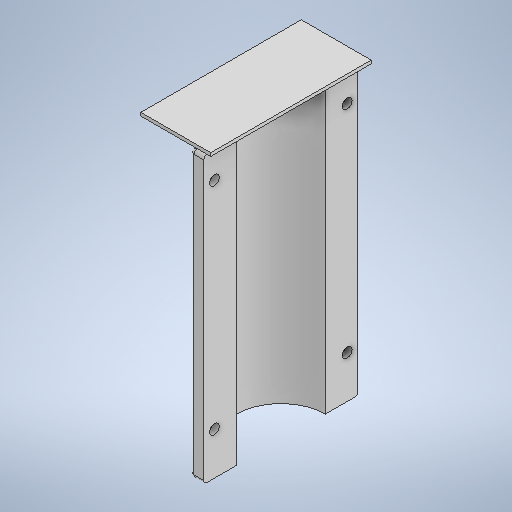
# Autodesk Inventor part: arm-2-2
Saved by Autodesk Inventor 2025.2 (Build 292293000, 293)
## iProperties
Created: 2025-02-07
Part Number: arm-2-2
Material: 一般
Document SubType Name: Modeling
Designer: mahhy
Density: 1 g/cm^3
Appearance: 既定
Author: mahhy
## iProperties of the stored document arm-2-2_3D プリント.ipt
Created: 2025-02-09
Part Number: arm-2-2_3D プリント
Material: 一般
Document SubType Name: Modeling
Designer: mahhy
Density: 1 g/cm^3
Appearance: 既定
Author: mahhy
Autodesk Inventor part; units mm, degrees
ref_plane "YZ Plane" through (0, 0, 0) normal (1, 0, 0) x (0, 1, 0)
ref_plane "XZ Plane" through (0, 0, 0) normal (0, 1, 0) x (-1, 0, 0)
ref_plane "XY Plane" through (0, 0, 0) normal (0, 0, 1) x (1, 0, 0)
sketch "スケッチ1" plane through (0, 0, 0) normal (0, 1, 0) x (-1, 0, 0)
  line L0 (0, 0) -> (20, 0)
  line L1 (20, 0) -> (20, -40)
  line L2 (20, -40) -> (0, -40)
  line L3 (0, -40) -> (0, 0)
  circle A0 centre (0, -20) radius 13.6
  circle A1 centre (0, -20) radius 17.5
  line L4 (0, -6.4) -> (4, -6.4)
  line L5 (4, -6.4) -> (4, 3.6)
  line L6 (4, 3.6) -> (0, 3.6)
  line L7 (0, 3.6) -> (0, -6.4)
  line L8 (0, -33.6) -> (4, -33.6)
  line L9 (4, -33.6) -> (4, -43.6)
  line L10 (4, -43.6) -> (0, -43.6)
  line L11 (0, -43.6) -> (0, -33.6)
  point P0 (0, -6.4)
  point P1 (0, -33.6)
  point P2 (4, -37.0367)
  point P3 (4, -2.9633)
  dimension "d0" = 20
  dimension "d1" = 40
  dimension "d2" = 27.2
  dimension "d3" = 35
  dimension "d4" = 4
  dimension "d5" = 10
  dimension "d6" = 4
  dimension "d7" = 10
  constraints: 24 end point, 6 parallel, 3 horizontal, 3 perpendicular, 2 centre point, 2 point on circle, 1 coincident, 1 midpoint
  measures "d0" distance of L1.end L2.end
  measures "d1" distance of L0.end L1.end
  measures "d2" diameter of A0
  measures "d3" diameter of A1
  measures "d4" distance of L6.end L5.end
  measures "d5" distance of L5.end L4.end
  measures "d6" distance of L9.end L10.end
  measures "d7" distance of L8.end L9.end
extrude "押し出し1" add sketch "スケッチ1" along normal blind 87 contours L7 L6 L5 L0 | L0 L5 A1 L3 | A1 L5 L4 L3 | A1 L9 L8 A0 L4 L5 | A1 L9 L2 L3 | L3 L8 L9 A1 | L2 L9 L10 L11
sketch "スケッチ2" plane through (-4, 0, -43.6) normal (-1, 0, 0) x (0, 0, 1)
  line L0 (0, 87) -> (6.5633, 87) projected
  line L1 (40.6367, 87) -> (47.2, 87) projected
  line L2 (40.6367, 0) -> (47.2, 0) projected
  line L3 (0, 0) -> (6.5633, 0) projected
  point P0 (43.6, 0)
  point P1 (3.2816, 13)
  point P2 (3.2816, 79)
  point P3 (43.9184, 79)
  point P4 (43.9184, 13)
  point P5 (3.2816, 87)
  point P6 (43.9184, 87)
  point P7 (43.9184, 0)
  point P8 (3.2816, 0)
  dimension "d10" = 0
  dimension "d11" = 8
  dimension "d12" = 0
  dimension "d13" = 8
  dimension "d14" = 0
  dimension "d15" = 0
  dimension "d16" = 13
  dimension "d17" = 13
  constraints: 4 midpoint
  measures "d10" horizontal distance of point (3.282, 87) point (3.282, 79)
  measures "d11" distance from line of L0 point (3.282, 79)
  measures "d12" horizontal distance of point (43.918, 87) point (43.918, 79)
  measures "d13" distance from line of L1 point (43.918, 79)
  measures "d14" horizontal distance of point (43.918, 0) point (43.918, 13)
  measures "d15" horizontal distance of point (3.282, 0) point (3.282, 13)
  measures "d16" vertical distance of L3.start point (3.282, 13)
  measures "d17" vertical distance of L2.end point (43.918, 13)
hole "穴1" at (-4, 13, -40.3184) at (-4, 79, -40.3184) at (-4, 79, 0.3184) at (-4, 13, 0.3184) direction (1, 0, 0) diameter 3 end through all
fillet "フィレット1" radius 1 14 edges at (-4, 87, 0.3184) (-17.5, 87, -20) (-4, 87, -40.3184) (-2, 87, -43.6) (-2, 87, 3.6) (-4, 43.5, 3.6) (-4, 0, 0.3184) (-17.5, 0, -20) (-4, 0, -40.3184) (-2, 0, -43.6) (-2, 0, 3.6) (-4, 43.5, -43.6) (-4, 43.5, -37.0367) (-4, 43.5, -2.9633)
sketch "スケッチ3" plane through (0, 87, 0) normal (0, 1, 0) x (1, 0, 0)
  line L0 (0, -2.6) -> (-3, -2.6) projected
  line L1 (-3, 42.6) -> (0, 42.6) projected
  circle A0 centre (-1.5, 39.6) radius 0.5
  circle A1 centre (-1.5, 0.4) radius 0.5
  circle A2 centre (-15.1647, 20) radius 0.5
  arc A3 (-4.7297, 36.8487) -> (-4.7297, 3.1513) centre (0, 20) ccw projected
  point P0 (-17.5, 20)
  dimension "d28" = 3
  dimension "d29" = 3
  dimension "d30" = 1
  dimension "d31" = 1
  dimension "d32" = 1
  dimension "d33" = 0
  constraints: 3 centre point, 3 coincident, 1 point on circle
  measures "d28" distance from line of L0 point (-1.5, 0.4)
  measures "d29" distance from line of L1 point (-1.5, 39.6)
  measures "d30" diameter of A0
  measures "d31" diameter of A1
  measures "d32" diameter of A2
  measures "d33" vertical distance of point (-17.5, 20) A2.centre
extrude "押し出し2" add sketch "スケッチ3" along normal blind 2
sketch "スケッチ4" plane through (-1.5, 89, -39.6) normal (0, 1, 0) x (1, 0, 0)
  line L0 (-16.7138, 4.8708) -> (4.6687, 4.8708)
  line L1 (4.6687, 4.8708) -> (4.6687, -44.2225)
  line L2 (4.6687, -44.2225) -> (-16.7138, -44.2225)
  line L3 (-16.7138, -44.2225) -> (-16.7138, 4.8708)
  point P0 (1.5, -39.6)
  constraints: 8 end point, 2 parallel, 1 horizontal, 1 perpendicular
extrude "押し出し3" add sketch "スケッチ4" along normal blind 1
sketch "スケッチ5" plane through (-4, 1, -37.8115) normal (-1, 0, 0) x (0, 0, 1)
  circle A0 centre (-2.5068, 12) radius 1.5 projected
  circle A1 centre (-2.5068, 12) radius 2.5
  circle A2 centre (38.1299, 12) radius 1.5 projected
  circle A3 centre (38.1299, 12) radius 2.5
  circle A4 centre (-2.5068, 78) radius 1.5 projected
  circle A5 centre (-2.5068, 78) radius 2.5
  circle A6 centre (38.1299, 78) radius 1.5 projected
  circle A7 centre (38.1299, 78) radius 2.5
  point P0 (37.8115, -1)
  dimension "d36" = 5
  dimension "d37" = 5
  dimension "d38" = 5
  dimension "d39" = 5
  constraints: 4 centre point, 4 coincident
  measures "d36" diameter of A1
  measures "d37" diameter of A3
  measures "d38" diameter of A5
  measures "d39" diameter of A7
extrude "押し出し4" cut sketch "スケッチ5" against normal blind 2
